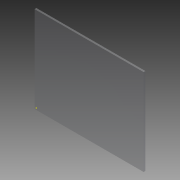
# Autodesk Inventor part: lateral
Saved by Autodesk Inventor 2015 (Build 190159000, 159)
## iProperties
Created: 2016-08-07
Part Number: lateral
Material: Polycarbonate, Clear
Document SubType Name: Modeling
Designer: Gabriel
Density: 1.2 g/cm^3
Appearance: Polycarbonate - Clear
Author: Gabriel
Autodesk Inventor part; units mm, degrees
ref_plane "YZ Plane" through (0, 0, 0) normal (1, 0, 0) x (0, 1, 0)
ref_plane "XZ Plane" through (0, 0, 0) normal (0, 1, 0) x (-1, 0, 0)
ref_plane "XY Plane" through (0, 0, 0) normal (0, 0, 1) x (1, 0, 0)
sketch "Sketch1" plane through (0, 0, 0) normal (0, 0, 1) x (1, 0, 0)
  point P0 (0, 0)
sketch "Sketch2" plane through (0, 0, 0) normal (0, 0, 1) x (1, 0, 0)
  line L0 (0, 0) -> (410, 0)
  line L1 (410, 0) -> (410, 325)
  line L2 (410, 325) -> (0, 325)
  line L3 (0, 325) -> (0, 0)
  dimension "d0" = 410
  dimension "d1" = 325
  constraints: 8 end point, 2 parallel, 1 horizontal, 1 perpendicular
  measures "d0" distance of L2.end L1.end
  measures "d1" distance of L1.end L0.end
extrude "Extrusion1" add sketch "Sketch2" along normal blind 7
body "Solid1"
